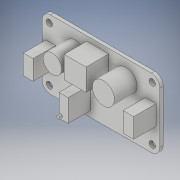
# Autodesk Inventor part: PowerSupply
Saved by Autodesk Inventor 2019.3 (Build 233278000, 278)
## iProperties
Created: 2019-02-11
Part Number: PowerSupply
Material: Generic
Document SubType Name: Modeling
Designer: mark
Density: 1 g/cm^3
Appearance: Default
Author: mark
Autodesk Inventor part; units mm, degrees
ref_plane "YZ Plane" through (0, 0, 0) normal (1, 0, 0) x (0, 1, 0)
ref_plane "XZ Plane" through (0, 0, 0) normal (0, 1, 0) x (-1, 0, 0)
ref_plane "XY Plane" through (0, 0, 0) normal (0, 0, 1) x (1, 0, 0)
sketch "Sketch1" plane through (0, 0, 0) normal (0, 0, 1) x (1, 0, 0)
  line L0 (0, 0) -> (55.5, 0)
  line L1 (55.5, 0) -> (55.5, 32.4)
  line L2 (55.5, 32.4) -> (0, 32.4)
  line L3 (0, 32.4) -> (0, 0)
  circle A0 centre (3.5, 28.9) radius 1.5
  circle A1 centre (52, 28.9) radius 1.5
  circle A2 centre (3.5, 3.5) radius 1.5
  circle A3 centre (52, 3.5) radius 1.5
  dimension "d0" = 55.5
  dimension "d1" = 32.4
  dimension "d2" = 3
  dimension "d3" = 3
  dimension "d4" = 3
  dimension "d5" = 3
  dimension "d6" = 3.5
  dimension "d7" = 3.5
  dimension "d8" = 3.5
  dimension "d9" = 3.5
  dimension "d10" = 3.5
  dimension "d11" = 3.5
  dimension "d12" = 3.5
  dimension "d13" = 3.5
  constraints: 8 end point, 4 centre point, 2 horizontal, 2 vertical
  measures "d0" distance between parallel lines of L1 L3
  measures "d1" distance between parallel lines of L0 L2
  measures "d2" diameter of A0
  measures "d3" diameter of A2
  measures "d4" diameter of A1
  measures "d5" diameter of A3
  measures "d6" distance from line of L3 A0.centre
  measures "d7" distance from line of L2 A0.centre
  measures "d8" distance from line of L3 A2.centre
  measures "d9" distance from line of L0 A2.centre
  measures "d10" distance from line of L2 A1.centre
  measures "d11" distance from line of L1 A1.centre
  measures "d12" distance from line of L1 A3.centre
  measures "d13" distance from line of L0 A3.centre
extrude "Extrusion1" add sketch "Sketch1" along normal blind 1.6
fillet "Fillet1" radius 4 4 edges at (55.5, 32.4, 0.8) (55.5, 0, 0.8) (0, 0, 0.8) (0, 32.4, 0.8)
sketch "Sketch2" plane through (0, 0, 1.6) normal (0, 0, 1) x (1, 0, 0)
  circle A0 centre (15.6251, 23.6367) radius 4.3835
  circle A1 centre (39.6101, 23.6367) radius 5.1943
  line L0 (1.8909, 21.1486) -> (6.469, 21.1486)
  line L1 (6.469, 21.1486) -> (6.469, 11.893)
  line L2 (6.469, 11.893) -> (1.8909, 11.893)
  line L3 (1.8909, 11.893) -> (1.8909, 21.1486)
  line L4 (48.8658, 21.1486) -> (53.8419, 21.1486)
  line L5 (53.8419, 21.1486) -> (53.8419, 11.893)
  line L6 (53.8419, 11.893) -> (48.8658, 11.893)
  line L7 (48.8658, 11.893) -> (48.8658, 21.1486)
  line L8 (21.0989, 30.2052) -> (31.4492, 30.2052)
  line L9 (31.4492, 30.2052) -> (31.4492, 19.8548)
  line L10 (31.4492, 19.8548) -> (21.0989, 19.8548)
  line L11 (21.0989, 19.8548) -> (21.0989, 30.2052)
  line L12 (18.7103, 13.4854) -> (22.9898, 13.4854)
  line L13 (22.9898, 13.4854) -> (22.9898, 2.9359)
  line L14 (22.9898, 2.9359) -> (18.7103, 2.9359)
  line L15 (18.7103, 2.9359) -> (18.7103, 13.4854)
  point P0 (0, 0)
  constraints: 32 end point, 2 centre point, 2 point on line
extrude "Extrusion2" add sketch "Sketch2" along normal blind 10.7
sketch "Sketch3" plane through (0, 0, 12.3) normal (0, 0, 1) x (1, 0, 0)
  circle A0 centre (19.5755, 4.3447) radius 0.7457
  point P0 (0, 0)
  constraints: 1 centre point
extrude "Extrusion3" add sketch "Sketch3" along normal blind 1.18
body "Solid1"
